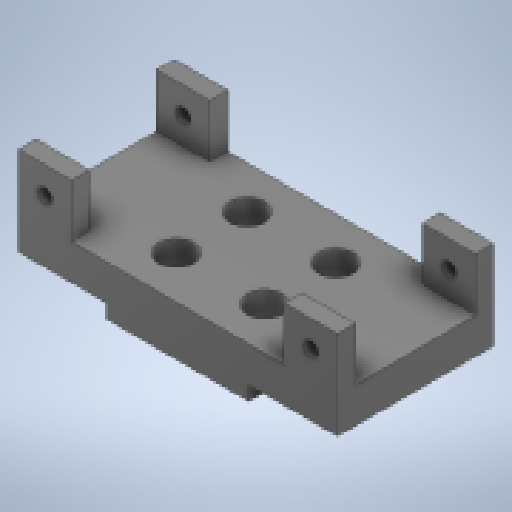
# Autodesk Inventor part: rail_top
Saved by Autodesk Inventor 2026.2 (Build 302298010, 298A)
## iProperties
Created: 2026-05-03
Part Number: rail_top
Material: ABS Plastic
Document SubType Name: Modeling
Designer: chris
Density: 1.06 g/cm^3
Appearance: Smooth - White
Author: chris
Autodesk Inventor part; units mm, degrees
ref_plane "YZ Plane" through (0, 0, 0) normal (1, 0, 0) x (0, 1, 0)
ref_plane "XZ Plane" through (0, 0, 0) normal (0, 1, 0) x (-1, 0, 0)
ref_plane "XY Plane" through (0, 0, 0) normal (0, 0, 1) x (1, 0, 0)
sketch "Sketch1" plane through (0, 0, 0) normal (0, 1, 0) x (-1, 0, 0)
  line L0 (45, 22) -> (-45, 22)
  line L1 (-45, 22) -> (-45, -22)
  line L2 (-45, -22) -> (45, -22)
  line L3 (45, -22) -> (45, 22)
  line L4 (45, 22) -> (-45, -22) construction
  line L5 (-45, 22) -> (45, -22) construction
  point P0 (0, 0)
  dimension "d0" = 90
  dimension "d1" = 44
  constraints: 12 end point, 2 midpoint, 2 parallel, 1 horizontal, 1 perpendicular
  measures "d0" distance of L2.end L1.end
  measures "d1" distance of L1.end L0.end
extrude "Extrusion1" add sketch "Sketch1" along normal blind 10
sketch "Sketch2" plane through (0, 10, 0) normal (0, 1, 0) x (1, 0, 0)
  line L0 (45, -22) -> (30, -22)
  line L1 (30, -22) -> (30, -17)
  line L2 (30, -17) -> (45, -17)
  line L3 (45, -17) -> (45, -22)
  line L4 (45, 17) -> (30, 17)
  line L5 (30, 17) -> (30, 22)
  line L6 (30, 22) -> (45, 22)
  line L7 (45, 22) -> (45, 17)
  line L8 (-45, -22) -> (-30, -22)
  line L9 (-30, -22) -> (-30, -17)
  line L10 (-30, -17) -> (-45, -17)
  line L11 (-45, -17) -> (-45, -22)
  line L12 (-45, 17) -> (-30, 17)
  line L13 (-30, 17) -> (-30, 22)
  line L14 (-30, 22) -> (-45, 22)
  line L15 (-45, 22) -> (-45, 17)
  line L16 (-45, 22) -> (-45, -22) projected
  line L17 (-45, -22) -> (45, -22) projected
  line L18 (45, 22) -> (-45, 22) projected
  line L19 (45, -22) -> (45, 22) projected
  point P0 (0, 0)
  dimension "d4" = 5
  dimension "d5" = 5
  dimension "d6" = 5
  dimension "d7" = 5
  dimension "d8" = 15
  dimension "d9" = 15
  dimension "d10" = 15
  dimension "d11" = 15
  constraints: 32 end point, 8 collinear, 8 parallel, 4 horizontal, 4 perpendicular
  measures "d4" distance of L2.end L0.start
  measures "d5" distance of L6.end L4.start
  measures "d6" distance of L12.end L13.end
  measures "d7" distance of L8.end L9.end
  measures "d8" distance of L0.start L0.end
  measures "d9" distance of L5.end L6.end
  measures "d10" distance of L12.start L12.end
  measures "d11" distance of L9.end L10.end
extrude "Extrusion2" add sketch "Sketch2" along normal blind 15 contours L0 L1 L2 L3 | L8 L11 L10 L9 | L4 L5 L6 L7 | L15 L14 L13 L12
sketch "Sketch3" plane through (-45, 0, 22) normal (0, 0, 1) x (1, 0, 0)
  circle A0 centre (82.5, 17.5) radius 2.05
  circle A1 centre (7.5, 17.5) radius 2.05
  line L0 (75, 25) -> (90, 25) projected
  line L1 (90, 0) -> (90, 25) projected
  line L2 (0, 25) -> (15, 25) projected
  line L3 (15, 10) -> (15, 25) projected
  point P0 (45, 0)
  point P1 (15, 17.5)
  dimension "d14" = 4.1
  dimension "d15" = 4.1
  dimension "d16" = 7.5
  dimension "d17" = 7.5
  dimension "d18" = 7.5
  dimension "d19" = 7.5
  constraints: 2 centre point, 1 midpoint
  measures "d14" diameter of A0
  measures "d15" diameter of A1
  measures "d16" distance from line of L0 A0.centre
  measures "d17" distance from line of L1 A0.centre
  measures "d18" distance from line of L2 A1.centre
  measures "d19" distance of point (15, 17.5) A1.centre
extrude "Extrusion3" cut sketch "Sketch3" against normal through all
sketch "Sketch4" plane through (0, 0, 0) normal (0, -1, 0) x (1, 0, 0)
  line L0 (-20, -22) -> (20, -22)
  line L1 (20, -22) -> (20, 22)
  line L2 (20, 22) -> (-20, 22)
  line L3 (-20, 22) -> (-20, -22)
  line L4 (-20, -22) -> (20, 22) construction
  line L5 (20, -22) -> (-20, 22) construction
  point P0 (0, 0)
  dimension "d22" = 40
  dimension "d23" = 44
  constraints: 12 end point, 2 midpoint, 2 parallel, 1 horizontal, 1 perpendicular
  measures "d22" distance of L2.end L1.end
  measures "d23" distance of L1.end L0.end
extrude "Extrusion4" add sketch "Sketch4" along normal blind 4
sketch "Sketch5" plane through (0, -4, 0) normal (0, -1, 0) x (1, 0, 0)
  circle A0 centre (-12.5, -10) radius 1.55
  circle A1 centre (12.5, -10) radius 1.55
  circle A2 centre (-12.5, 10) radius 1.55
  circle A3 centre (12.5, 10) radius 1.55
  point P0 (0, 0)
  dimension "d26" = 3.1
  dimension "d27" = 3.1
  dimension "d28" = 3.1
  dimension "d29" = 3.1
  dimension "d30" = 12.5
  dimension "d31" = 12.5
  dimension "d32" = 12.5
  dimension "d33" = 12.5
  dimension "d34" = 10
  dimension "d35" = 10
  dimension "d36" = 10
  dimension "d37" = 10
  constraints: 4 centre point
  measures "d26" diameter of A0
  measures "d27" diameter of A1
  measures "d28" diameter of A2
  measures "d29" diameter of A3
  measures "d30" horizontal distance of A0.centre point (0, 0)
  measures "d31" horizontal distance of point (0, 0) A1.centre
  measures "d32" horizontal distance of point (0, 0) A3.centre
  measures "d33" horizontal distance of A2.centre point (0, 0)
  measures "d34" vertical distance of point (0, 0) A1.centre
  measures "d35" vertical distance of point (0, 0) A3.centre
  measures "d36" vertical distance of A0.centre point (0, 0)
  measures "d37" vertical distance of A2.centre point (0, 0)
extrude "Extrusion5" cut sketch "Sketch5" against normal through all
sketch "Sketch6" plane through (0, 10, 0) normal (0, 1, 0) x (1, 0, 0)
  circle A0 centre (12.5, -10) radius 1.55 projected
  circle A1 centre (-12.5, -10) radius 1.55 projected
  circle A2 centre (12.5, 10) radius 1.55 projected
  circle A3 centre (-12.5, 10) radius 1.55 projected
  circle A4 centre (12.5, -10) radius 5
  circle A5 centre (-12.5, -10) radius 5
  circle A6 centre (12.5, 10) radius 5
  circle A7 centre (-12.5, 10) radius 5
  point P0 (0, 0)
  dimension "d40" = 10
  dimension "d41" = 10
  dimension "d42" = 10
  dimension "d43" = 10
  constraints: 4 centre point, 4 coincident
  measures "d40" diameter of A4
  measures "d41" diameter of A5
  measures "d42" diameter of A6
  measures "d43" diameter of A7
extrude "Extrusion6" cut sketch "Sketch6" against normal blind 7
body "Solid1"
